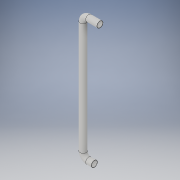
# Autodesk Inventor part: connector2
Saved by Autodesk Inventor 2017 (Build 210142000, 142)
## iProperties
Created: 2017-02-09
Part Number: connector2
Material: Generic
Document SubType Name: Modeling
Designer: XuZhiqing
Density: 1 g/cm^3
Appearance: Default
Author: XuZhiqing
Autodesk Inventor part; units mm, degrees
ref_plane "YZ Plane" through (0, 0, 0) normal (1, 0, 0) x (0, 1, 0)
ref_plane "XZ Plane" through (0, 0, 0) normal (0, 1, 0) x (-1, 0, 0)
ref_plane "XY Plane" through (0, 0, 0) normal (0, 0, 1) x (1, 0, 0)
sketch "Sketch2" plane through (0, 0, 0) normal (0, 0, 1) x (1, 0, 0)
  line L0 (0, 0) -> (-50.8, 0)
  line L1 (-101.6, 50.8) -> (-101.6, 1066.8)
  line L2 (-50.8, 1117.6) -> (50.8, 1117.6)
  arc A0 (-50.8, 1117.6) -> (-101.6, 1066.8) centre (-50.8, 1066.8) ccw
  arc A1 (-101.6, 50.8) -> (-50.8, 0) centre (-50.8, 50.8) ccw
  point P0 (0, 1117.6)
  dimension "d1" = 50.8
  dimension "d3" = 1016
  dimension "d6" = 101.6
  dimension "d7" = 101.6
  dimension "d8" = 50.8
  dimension "d9" = 1117.6
  dimension "d10" = 50.8
  dimension "d11" = 50.8
  dimension "d12" = 50.8
  constraints: 6 end point, 4 point on circle, 2 centre point, 1 horizontal, 1 midpoint, 1 vertical, 1 vertical alignment
  measures "d1" distance of L0.start L0.end
  measures "d3" distance of L1.start L1.end
  measures "d6" distance of L2.start L2.end
  measures "d7" distance from line of L0.start L1
  measures "d8" vertical distance of L0.start L1.start
  measures "d9" vertical distance of L0.start L2.start
  measures "d10" distance of point (0, 1117.6) L2.start
  measures "d11" radius of A0
  measures "d12" radius of A1
sketch "Sketch3" plane through (0, 0, 0) normal (1, 0, 0) x (0, 1, 0)
  circle A0 centre (0, 0) radius 27.94
  dimension "d13" = 55.88
  constraints: 1 centre point, 1 coincident
  measures "d13" diameter of A0
sweep "Sweep1" add profiles "Sketch3" path "Sketch2"
shell "Shell1" thickness 2.54 removed faces 2 at (0, -1.1226, -9.2454) at (50.8, 1125.8465, -0.1295)
body "Solid1"
